Autodesk Inventor part; units mm, degrees
note: some values were not read from the file. Chosen so that the rebuilt part matches the saved one: sketch regions of "Extrusion1".
(part 2 of 2)
sketch "Sketch2" plane through (0, 0, 0) normal (0, -1, 0) x (1, 0, 0)
  line L0 (-1.935, 1.0367) -> (-1.9383, 1.036) projected
  line L1 (-1.9383, 1.036) -> (-1.9449, 1.0346) projected
  line L2 (-1.9449, 1.0346) -> (-1.9582, 1.0311) projected
  line L3 (-1.9582, 1.0311) -> (-1.9714, 1.0269) projected
  line L4 (-1.9714, 1.0269) -> (-1.9846, 1.0221) projected
  line L5 (-1.9846, 1.0221) -> (-1.9978, 1.0168) projected
  line L6 (-1.9978, 1.0168) -> (-2.0109, 1.0108) projected
  line L7 (-2.0109, 1.0108) -> (-2.0098, 0.9593) projected
  line L8 (-2.0098, 0.9593) -> (-1.9964, 0.9539) projected
  line L9 (-1.9964, 0.9539) -> (-1.983, 0.9491) projected
  line L10 (-1.983, 0.9491) -> (-1.9696, 0.9449) projected
  line L11 (-1.9696, 0.9449) -> (-1.9562, 0.9412) projected
  line L12 (-1.9562, 0.9412) -> (-1.9429, 0.9383) projected
  line L13 (-1.9429, 0.9383) -> (-1.9362, 0.9371) projected
  line L14 (-1.9362, 0.9371) -> (-1.9329, 0.9366) projected
  line L15 (-1.9329, 0.9366) -> (-1.9296, 0.9361) projected
  line L16 (-1.9296, 0.9361) -> (-1.9237, 0.8803) projected
  line L17 (-1.9237, 0.8803) -> (-1.9268, 0.8792) projected
  line L18 (-1.9268, 0.8792) -> (-1.93, 0.878) projected
  line L19 (-1.93, 0.878) -> (-1.9363, 0.8754) projected
  line L20 (-1.9363, 0.8754) -> (-1.9487, 0.8698) projected
  line L21 (-1.9487, 0.8698) -> (-1.961, 0.8634) projected
  line L22 (-1.961, 0.8634) -> (-1.9732, 0.8565) projected
  line L23 (-1.9732, 0.8565) -> (-1.9853, 0.849) projected
  line L24 (-1.9853, 0.849) -> (-1.9973, 0.8409) projected
  line L25 (-1.9973, 0.8409) -> (-1.9876, 0.7902) projected
  line L26 (-1.9876, 0.7902) -> (-1.9735, 0.7872) projected
  line L27 (-1.9735, 0.7872) -> (-1.9595, 0.7847) projected
  line L28 (-1.9595, 0.7847) -> (-1.9455, 0.7828) projected
  line L29 (-1.9455, 0.7828) -> (-1.9317, 0.7815) projected
  line L30 (-1.9317, 0.7815) -> (-1.9181, 0.7808) projected
  line L31 (-1.9181, 0.7808) -> (-1.9113, 0.7808) projected
  line L32 (-1.9113, 0.7808) -> (-1.9079, 0.7808) projected
  line L33 (-1.9079, 0.7808) -> (-1.9046, 0.7809) projected
  line L34 (-1.9046, 0.7809) -> (-1.8893, 0.727) projected
  line L35 (-1.8893, 0.727) -> (-1.8923, 0.7253) projected
  line L36 (-1.8923, 0.7253) -> (-1.8952, 0.7236) projected
  line L37 (-1.8952, 0.7236) -> (-1.9009, 0.72) projected
  line L38 (-1.9009, 0.72) -> (-1.9122, 0.7123) projected
  line L39 (-1.9122, 0.7123) -> (-1.9233, 0.704) projected
  line L40 (-1.9233, 0.704) -> (-1.9342, 0.6951) projected
  line L41 (-1.9342, 0.6951) -> (-1.9448, 0.6856) projected
  line L42 (-1.9448, 0.6856) -> (-1.9553, 0.6757) projected
  line L43 (-1.9553, 0.6757) -> (-1.9371, 0.6273) projected
  line L44 (-1.9371, 0.6273) -> (-1.9226, 0.6267) projected
  line L45 (-1.9226, 0.6267) -> (-1.9084, 0.6267) projected
  line L46 (-1.9084, 0.6267) -> (-1.8944, 0.6271) projected
  line L47 (-1.8944, 0.6271) -> (-1.8805, 0.6282) projected
  line L48 (-1.8805, 0.6282) -> (-1.8669, 0.6298) projected
  line L49 (-1.8669, 0.6298) -> (-1.8603, 0.6309) projected
  line L50 (-1.8603, 0.6309) -> (-1.857, 0.6316) projected
  line L51 (-1.857, 0.6316) -> (-1.8537, 0.6322) projected
  line L52 (-1.8537, 0.6322) -> (-1.8295, 0.5816) projected
  line L53 (-1.8295, 0.5816) -> (-1.8321, 0.5795) projected
  line L54 (-1.8321, 0.5795) -> (-1.8347, 0.5773) projected
  line L55 (-1.8347, 0.5773) -> (-1.8397, 0.5728) projected
  line L56 (-1.8397, 0.5728) -> (-1.8496, 0.5633) projected
  line L57 (-1.8496, 0.5633) -> (-1.8591, 0.5532) projected
  line L58 (-1.8591, 0.5532) -> (-1.8683, 0.5426) projected
  line L59 (-1.8683, 0.5426) -> (-1.8772, 0.5315) projected
  line L60 (-1.8772, 0.5315) -> (-1.8858, 0.5199) projected
  line L61 (-1.8858, 0.5199) -> (-1.8597, 0.4753) projected
  line L62 (-1.8597, 0.4753) -> (-1.8454, 0.4772) projected
  line L63 (-1.8454, 0.4772) -> (-1.8314, 0.4795) projected
  line L64 (-1.8314, 0.4795) -> (-1.8176, 0.4823) projected
  line L65 (-1.8176, 0.4823) -> (-1.8042, 0.4857) projected
  line L66 (-1.8042, 0.4857) -> (-1.7911, 0.4896) projected
  line L67 (-1.7911, 0.4896) -> (-1.7847, 0.4919) projected
  line L68 (-1.7847, 0.4919) -> (-1.7815, 0.493) projected
  line L69 (-1.7815, 0.493) -> (-1.7784, 0.4942) projected
  line L70 (-1.7784, 0.4942) -> (-1.746, 0.4484) projected
  line L71 (-1.746, 0.4484) -> (-1.7482, 0.4459) projected
  line L72 (-1.7482, 0.4459) -> (-1.7504, 0.4433) projected
  line L73 (-1.7504, 0.4433) -> (-1.7546, 0.438) projected
  line L74 (-1.7546, 0.438) -> (-1.7627, 0.427) projected
  line L75 (-1.7627, 0.427) -> (-1.7704, 0.4154) projected
  line L76 (-1.7704, 0.4154) -> (-1.7776, 0.4034) projected
  line L77 (-1.7776, 0.4034) -> (-1.7845, 0.391) projected
  line L78 (-1.7845, 0.391) -> (-1.7911, 0.3781) projected
  line L79 (-1.7911, 0.3781) -> (-1.7578, 0.3386) projected
  line L80 (-1.7578, 0.3386) -> (-1.744, 0.3428) projected
  line L81 (-1.744, 0.3428) -> (-1.7306, 0.3475) projected
  line L82 (-1.7306, 0.3475) -> (-1.7175, 0.3526) projected
  line L83 (-1.7175, 0.3526) -> (-1.7048, 0.3582) projected
  line L84 (-1.7048, 0.3582) -> (-1.6926, 0.3643) projected
  line L85 (-1.6926, 0.3643) -> (-1.6866, 0.3676) projected
  line L86 (-1.6866, 0.3676) -> (-1.6837, 0.3692) projected
  line L87 (-1.6837, 0.3692) -> (-1.6808, 0.371) projected
  line L88 (-1.6808, 0.371) -> (-1.6412, 0.3313) projected
  line L89 (-1.6412, 0.3313) -> (-1.6429, 0.3284) projected
  line L90 (-1.6429, 0.3284) -> (-1.6446, 0.3255) projected
  line L91 (-1.6446, 0.3255) -> (-1.6479, 0.3196) projected
  line L92 (-1.6479, 0.3196) -> (-1.654, 0.3073) projected
  line L93 (-1.654, 0.3073) -> (-1.6596, 0.2947) projected
  line L94 (-1.6596, 0.2947) -> (-1.6648, 0.2816) projected
  line L95 (-1.6648, 0.2816) -> (-1.6695, 0.2681) projected
  line L96 (-1.6695, 0.2681) -> (-1.6737, 0.2543) projected
  line L97 (-1.6737, 0.2543) -> (-1.6343, 0.221) projected
  line L98 (-1.6343, 0.221) -> (-1.6214, 0.2275) projected
  line L99 (-1.6214, 0.2275) -> (-1.6089, 0.2344) projected
  line L100 (-1.6089, 0.2344) -> (-1.5969, 0.2417) projected
  line L101 (-1.5969, 0.2417) -> (-1.5853, 0.2493) projected
  line L102 (-1.5853, 0.2493) -> (-1.5743, 0.2574) projected
  line L103 (-1.5743, 0.2574) -> (-1.569, 0.2616) projected
  line L104 (-1.569, 0.2616) -> (-1.5664, 0.2638) projected
  line L105 (-1.5664, 0.2638) -> (-1.5639, 0.266) projected
  line L106 (-1.5639, 0.266) -> (-1.5181, 0.2335) projected
  line L107 (-1.5181, 0.2335) -> (-1.5193, 0.2304) projected
  line L108 (-1.5193, 0.2304) -> (-1.5205, 0.2273) projected
  line L109 (-1.5205, 0.2273) -> (-1.5227, 0.2209) projected
  line L110 (-1.5227, 0.2209) -> (-1.5267, 0.2078) projected
  line L111 (-1.5267, 0.2078) -> (-1.5301, 0.1943) projected
  line L112 (-1.5301, 0.1943) -> (-1.5329, 0.1806) projected
  line L113 (-1.5329, 0.1806) -> (-1.5353, 0.1665) projected
  line L114 (-1.5353, 0.1665) -> (-1.5372, 0.1522) projected
  line L115 (-1.5372, 0.1522) -> (-1.4927, 0.126) projected
  line L116 (-1.4927, 0.126) -> (-1.4811, 0.1346) projected
  line L117 (-1.4811, 0.1346) -> (-1.4699, 0.1435) projected
  line L118 (-1.4699, 0.1435) -> (-1.4593, 0.1527) projected
  line L119 (-1.4593, 0.1527) -> (-1.4492, 0.1622) projected
  line L120 (-1.4492, 0.1622) -> (-1.4397, 0.172) projected
  line L121 (-1.4397, 0.172) -> (-1.4352, 0.1771) projected
  line L122 (-1.4352, 0.1771) -> (-1.433, 0.1796) projected
  line L123 (-1.433, 0.1796) -> (-1.4309, 0.1822) projected
  line L124 (-1.4309, 0.1822) -> (-1.3803, 0.158) projected
  line L125 (-1.3803, 0.158) -> (-1.3809, 0.1547) projected
  line L126 (-1.3809, 0.1547) -> (-1.3816, 0.1514) projected
  line L127 (-1.3816, 0.1514) -> (-1.3827, 0.1447) projected
  line L128 (-1.3827, 0.1447) -> (-1.3844, 0.1312) projected
  line L129 (-1.3844, 0.1312) -> (-1.3854, 0.1173) projected
  line L130 (-1.3854, 0.1173) -> (-1.3859, 0.1033) projected
  line L131 (-1.3859, 0.1033) -> (-1.3859, 0.089) projected
  line L132 (-1.3859, 0.089) -> (-1.3853, 0.0746) projected
  line L133 (-1.3853, 0.0746) -> (-1.337, 0.0563) projected
  line L134 (-1.337, 0.0563) -> (-1.327, 0.0668) projected
  line L135 (-1.327, 0.0668) -> (-1.3176, 0.0774) projected
  line L136 (-1.3176, 0.0774) -> (-1.3086, 0.0883) projected
  line L137 (-1.3086, 0.0883) -> (-1.3003, 0.0993) projected
  line L138 (-1.3003, 0.0993) -> (-1.2926, 0.1106) projected
  line L139 (-1.2926, 0.1106) -> (-1.289, 0.1164) projected
  line L140 (-1.289, 0.1164) -> (-1.2873, 0.1193) projected
  line L141 (-1.2873, 0.1193) -> (-1.2856, 0.1222) projected
  line L142 (-1.2856, 0.1222) -> (-1.2316, 0.1068) projected
  line L143 (-1.2316, 0.1068) -> (-1.2318, 0.1035) projected
  line L144 (-1.2318, 0.1035) -> (-1.2318, 0.1001) projected
  line L145 (-1.2318, 0.1001) -> (-1.2318, 0.0934) projected
  line L146 (-1.2318, 0.0934) -> (-1.2312, 0.0797) projected
  line L147 (-1.2312, 0.0797) -> (-1.2299, 0.0659) projected
  line L148 (-1.2299, 0.0659) -> (-1.228, 0.052) projected
  line L149 (-1.228, 0.052) -> (-1.2255, 0.0379) projected
  line L150 (-1.2255, 0.0379) -> (-1.2225, 0.0238) projected
  line L151 (-1.2225, 0.0238) -> (-1.1718, 0.014) projected
  line L152 (-1.1718, 0.014) -> (-1.1638, 0.0259) projected
  line L153 (-1.1638, 0.0259) -> (-1.1562, 0.038) projected
  line L154 (-1.1562, 0.038) -> (-1.1492, 0.0502) projected
  line L155 (-1.1492, 0.0502) -> (-1.1429, 0.0625) projected
  line L156 (-1.1429, 0.0625) -> (-1.1372, 0.075) projected
  line L157 (-1.1372, 0.075) -> (-1.1346, 0.0812) projected
  line L158 (-1.1346, 0.0812) -> (-1.1334, 0.0844) projected
  line L159 (-1.1334, 0.0844) -> (-1.1323, 0.0875) projected
  line L160 (-1.1323, 0.0875) -> (-1.0765, 0.0815) projected
  line L161 (-1.0765, 0.0815) -> (-1.076, 0.0782) projected
  line L162 (-1.076, 0.0782) -> (-1.0755, 0.0749) projected
  line L163 (-1.0755, 0.0749) -> (-1.0744, 0.0682) projected
  line L164 (-1.0744, 0.0682) -> (-1.0714, 0.0548) projected
  line L165 (-1.0714, 0.0548) -> (-1.0678, 0.0415) projected
  line L166 (-1.0678, 0.0415) -> (-1.0636, 0.028) projected
  line L167 (-1.0636, 0.028) -> (-1.0588, 0.0146) projected
  line L168 (-1.0588, 0.0146) -> (-1.0535, 0.0012) projected
  line L169 (-1.0535, 0.0012) -> (-1.0019, 0.0001) projected
  line L170 (-1.0019, 0.0001) -> (-0.9959, 0.0132) projected
  line L171 (-0.9959, 0.0132) -> (-0.9905, 0.0264) projected
  line L172 (-0.9905, 0.0264) -> (-0.9857, 0.0396) projected
  line L173 (-0.9857, 0.0396) -> (-0.9815, 0.0528) projected
  line L174 (-0.9815, 0.0528) -> (-0.978, 0.0661) projected
  line L175 (-0.978, 0.0661) -> (-0.9765, 0.0727) projected
  line L176 (-0.9765, 0.0727) -> (-0.9759, 0.076) projected
  line L177 (-0.9759, 0.076) -> (-0.9753, 0.0793) projected
  line L178 (-0.9753, 0.0793) -> (-0.9193, 0.0828) projected
  line L179 (-0.9193, 0.0828) -> (-0.9183, 0.0796) projected
  line L180 (-0.9183, 0.0796) -> (-0.9172, 0.0764) projected
  line L181 (-0.9172, 0.0764) -> (-0.9149, 0.07) projected
  line L182 (-0.9149, 0.07) -> (-0.9098, 0.0573) projected
  line L183 (-0.9098, 0.0573) -> (-0.904, 0.0448) projected
  line L184 (-0.904, 0.0448) -> (-0.8976, 0.0323) projected
  line L185 (-0.8976, 0.0323) -> (-0.8906, 0.0198) projected
  line L186 (-0.8906, 0.0198) -> (-0.883, 0.0075) projected
  line L187 (-0.883, 0.0075) -> (-0.832, 0.0151) projected
  line L188 (-0.832, 0.0151) -> (-0.8284, 0.0291) projected
  line L189 (-0.8284, 0.0291) -> (-0.8253, 0.043) projected
  line L190 (-0.8253, 0.043) -> (-0.8228, 0.0568) projected
  line L191 (-0.8228, 0.0568) -> (-0.8209, 0.0706) projected
  line L192 (-0.8209, 0.0706) -> (-0.8197, 0.0842) projected
  line L193 (-0.8197, 0.0842) -> (-0.8193, 0.0909) projected
  line L194 (-0.8193, 0.0909) -> (-0.8192, 0.0943) projected
  line L195 (-0.8192, 0.0943) -> (-0.8192, 0.0977) projected
  line L196 (-0.8192, 0.0977) -> (-0.7646, 0.1106) projected
  line L197 (-0.7646, 0.1106) -> (-0.7631, 0.1076) projected
  line L198 (-0.7631, 0.1076) -> (-0.7615, 0.1046) projected
  line L199 (-0.7615, 0.1046) -> (-0.7581, 0.0987) projected
  line L200 (-0.7581, 0.0987) -> (-0.751, 0.0871) projected
  line L201 (-0.751, 0.0871) -> (-0.7431, 0.0757) projected
  line L202 (-0.7431, 0.0757) -> (-0.7347, 0.0645) projected
  line L203 (-0.7347, 0.0645) -> (-0.7257, 0.0534) projected
  line L204 (-0.7257, 0.0534) -> (-0.7161, 0.0426) projected
  line L205 (-0.7161, 0.0426) -> (-0.6671, 0.0587) projected
  line L206 (-0.6671, 0.0587) -> (-0.6659, 0.0731) projected
  line L207 (-0.6659, 0.0731) -> (-0.6652, 0.0873) projected
  line L208 (-0.6652, 0.0873) -> (-0.6651, 0.1013) projected
  line L209 (-0.6651, 0.1013) -> (-0.6655, 0.1152) projected
  line L210 (-0.6655, 0.1152) -> (-0.6666, 0.1288) projected
  line L211 (-0.6666, 0.1288) -> (-0.6674, 0.1355) projected
  line L212 (-0.6674, 0.1355) -> (-0.6679, 0.1389) projected
  line L213 (-0.6679, 0.1389) -> (-0.6684, 0.1422) projected
  line L214 (-0.6684, 0.1422) -> (-0.6168, 0.1641) projected
  line L215 (-0.6168, 0.1641) -> (-0.6148, 0.1615) projected
  line L216 (-0.6148, 0.1615) -> (-0.6127, 0.1588) projected
  line L217 (-0.6127, 0.1588) -> (-0.6085, 0.1536) projected
  line L218 (-0.6085, 0.1536) -> (-0.5994, 0.1433) projected
  line L219 (-0.5994, 0.1433) -> (-0.5897, 0.1334) projected
  line L220 (-0.5897, 0.1334) -> (-0.5795, 0.1238) projected
  line L221 (-0.5795, 0.1238) -> (-0.5688, 0.1144) projected
  line L222 (-0.5688, 0.1144) -> (-0.5576, 0.1053) projected
  line L223 (-0.5576, 0.1053) -> (-0.512, 0.1294) projected
  line L224 (-0.512, 0.1294) -> (-0.5132, 0.1438) projected
  line L225 (-0.5132, 0.1438) -> (-0.5149, 0.158) projected
  line L226 (-0.5149, 0.158) -> (-0.5172, 0.1718) projected
  line L227 (-0.5172, 0.1718) -> (-0.5199, 0.1854) projected
  line L228 (-0.5199, 0.1854) -> (-0.5233, 0.1987) projected
  line L229 (-0.5233, 0.1987) -> (-0.5253, 0.2052) projected
  line L230 (-0.5253, 0.2052) -> (-0.5263, 0.2084) projected
  line L231 (-0.5263, 0.2084) -> (-0.5274, 0.2115) projected
  line L232 (-0.5274, 0.2115) -> (-0.4802, 0.2419) projected
  line L233 (-0.4802, 0.2419) -> (-0.4778, 0.2396) projected
  line L234 (-0.4778, 0.2396) -> (-0.4753, 0.2373) projected
  line L235 (-0.4753, 0.2373) -> (-0.4702, 0.2329) projected
  line L236 (-0.4702, 0.2329) -> (-0.4595, 0.2243) projected
  line L237 (-0.4595, 0.2243) -> (-0.4483, 0.2162) projected
  line L238 (-0.4483, 0.2162) -> (-0.4366, 0.2084) projected
  line L239 (-0.4366, 0.2084) -> (-0.4244, 0.201) projected
  line L240 (-0.4244, 0.201) -> (-0.4119, 0.1939) projected
  line L241 (-0.4119, 0.1939) -> (-0.371, 0.2254) projected
  line L242 (-0.371, 0.2254) -> (-0.3746, 0.2394) projected
  line L243 (-0.3746, 0.2394) -> (-0.3787, 0.2531) projected
  line L244 (-0.3787, 0.2531) -> (-0.3833, 0.2664) projected
  line L245 (-0.3833, 0.2664) -> (-0.3883, 0.2793) projected
  line L246 (-0.3883, 0.2793) -> (-0.3939, 0.2918) projected
  line L247 (-0.3939, 0.2918) -> (-0.3969, 0.2978) projected
  line L248 (-0.3969, 0.2978) -> (-0.3985, 0.3008) projected
  line L249 (-0.3985, 0.3008) -> (-0.4001, 0.3037) projected
  line L250 (-0.4001, 0.3037) -> (-0.3587, 0.3417) projected
  line L251 (-0.3587, 0.3417) -> (-0.3559, 0.3398) projected
  line L252 (-0.3559, 0.3398) -> (-0.3531, 0.338) projected
  line L253 (-0.3531, 0.338) -> (-0.3473, 0.3345) projected
  line L254 (-0.3473, 0.3345) -> (-0.3354, 0.3278) projected
  line L255 (-0.3354, 0.3278) -> (-0.3229, 0.3217) projected
  line L256 (-0.3229, 0.3217) -> (-0.3101, 0.316) projected
  line L257 (-0.3101, 0.316) -> (-0.2969, 0.3108) projected
  line L258 (-0.2969, 0.3108) -> (-0.2832, 0.3059) projected
  line L259 (-0.2832, 0.3059) -> (-0.2483, 0.3439) projected
  line L260 (-0.2483, 0.3439) -> (-0.2543, 0.357) projected
  line L261 (-0.2543, 0.357) -> (-0.2606, 0.3698) projected
  line L262 (-0.2606, 0.3698) -> (-0.2673, 0.3821) projected
  line L263 (-0.2673, 0.3821) -> (-0.2745, 0.394) projected
  line L264 (-0.2745, 0.394) -> (-0.2821, 0.4054) projected
  line L265 (-0.2821, 0.4054) -> (-0.2861, 0.4108) projected
  line L266 (-0.2861, 0.4108) -> (-0.2881, 0.4135) projected
  line L267 (-0.2881, 0.4135) -> (-0.2902, 0.4161) projected
  line L268 (-0.2902, 0.4161) -> (-0.2559, 0.4605) projected
  line L269 (-0.2559, 0.4605) -> (-0.2528, 0.4592) projected
  line L270 (-0.2528, 0.4592) -> (-0.2497, 0.4578) projected
  line L271 (-0.2497, 0.4578) -> (-0.2434, 0.4553) projected
  line L272 (-0.2434, 0.4553) -> (-0.2305, 0.4508) projected
  line L273 (-0.2305, 0.4508) -> (-0.2172, 0.4469) projected
  line L274 (-0.2172, 0.4469) -> (-0.2036, 0.4434) projected
  line L275 (-0.2036, 0.4434) -> (-0.1896, 0.4405) projected
  line L276 (-0.1896, 0.4405) -> (-0.1754, 0.438) projected
  line L277 (-0.1754, 0.438) -> (-0.1474, 0.4814) projected
  line L278 (-0.1474, 0.4814) -> (-0.1555, 0.4933) projected
  line L279 (-0.1555, 0.4933) -> (-0.1639, 0.5048) projected
  line L280 (-0.1639, 0.5048) -> (-0.1726, 0.5158) projected
  line L281 (-0.1726, 0.5158) -> (-0.1817, 0.5263) projected
  line L282 (-0.1817, 0.5263) -> (-0.1911, 0.5363) projected
  line L283 (-0.1911, 0.5363) -> (-0.1959, 0.541) projected
  line L284 (-0.1959, 0.541) -> (-0.1984, 0.5433) projected
  line L285 (-0.1984, 0.5433) -> (-0.2009, 0.5455) projected
  line L286 (-0.2009, 0.5455) -> (-0.1745, 0.595) projected
  line L287 (-0.1745, 0.595) -> (-0.1713, 0.5942) projected
  line L288 (-0.1713, 0.5942) -> (-0.168, 0.5934) projected
  line L289 (-0.168, 0.5934) -> (-0.1614, 0.592) projected
  line L290 (-0.1614, 0.592) -> (-0.1479, 0.5898) projected
  line L291 (-0.1479, 0.5898) -> (-0.1341, 0.5881) projected
  line L292 (-0.1341, 0.5881) -> (-0.1201, 0.587) projected
  line L293 (-0.1201, 0.587) -> (-0.1059, 0.5865) projected
  line L294 (-0.1059, 0.5865) -> (-0.0915, 0.5865) projected
  line L295 (-0.0915, 0.5865) -> (-0.0712, 0.6339) projected
  line L296 (-0.0712, 0.6339) -> (-0.0812, 0.6443) projected
  line L297 (-0.0812, 0.6443) -> (-0.0914, 0.6543) projected
  line L298 (-0.0914, 0.6543) -> (-0.1018, 0.6636) projected
  line L299 (-0.1018, 0.6636) -> (-0.1125, 0.6725) projected
  line L300 (-0.1125, 0.6725) -> (-0.1235, 0.6806) projected
  line L301 (-0.1235, 0.6806) -> (-0.1291, 0.6845) projected
  line L302 (-0.1291, 0.6845) -> (-0.1319, 0.6863) projected
  line L303 (-0.1319, 0.6863) -> (-0.1347, 0.6881) projected
  line L304 (-0.1347, 0.6881) -> (-0.1171, 0.7414) projected
  line L305 (-0.1171, 0.7414) -> (-0.1138, 0.7411) projected
  line L306 (-0.1138, 0.7411) -> (-0.1104, 0.7409) projected
  line L307 (-0.1104, 0.7409) -> (-0.1037, 0.7406) projected
  line L308 (-0.1037, 0.7406) -> (-0.09, 0.7407) projected
  line L309 (-0.09, 0.7407) -> (-0.0761, 0.7414) projected
  line L310 (-0.0761, 0.7414) -> (-0.0621, 0.7427) projected
  line L311 (-0.0621, 0.7427) -> (-0.048, 0.7446) projected
  line L312 (-0.048, 0.7446) -> (-0.0338, 0.747) projected
  line L313 (-0.0338, 0.747) -> (-0.0218, 0.7972) projected
  line L314 (-0.0218, 0.7972) -> (-0.0334, 0.8057) projected
  line L315 (-0.0334, 0.8057) -> (-0.0452, 0.8138) projected
  line L316 (-0.0452, 0.8138) -> (-0.0571, 0.8213) projected
  line L317 (-0.0571, 0.8213) -> (-0.0691, 0.8282) projected
  line L318 (-0.0691, 0.8282) -> (-0.0813, 0.8344) projected
  line L319 (-0.0813, 0.8344) -> (-0.0874, 0.8372) projected
  line L320 (-0.0874, 0.8372) -> (-0.0905, 0.8385) projected
  line L321 (-0.0905, 0.8385) -> (-0.0936, 0.8398) projected
  line L322 (-0.0936, 0.8398) -> (-0.0853, 0.8953) projected
  line L323 (-0.0853, 0.8953) -> (-0.0819, 0.8956) projected
  line L324 (-0.0819, 0.8956) -> (-0.0786, 0.896) projected
  line L325 (-0.0786, 0.896) -> (-0.0719, 0.8969) projected
  line L326 (-0.0719, 0.8969) -> (-0.0584, 0.8992) projected
  line L327 (-0.0584, 0.8992) -> (-0.0449, 0.9022) projected
  line L328 (-0.0449, 0.9022) -> (-0.0313, 0.9059) projected
  line L329 (-0.0313, 0.9059) -> (-0.0177, 0.9101) projected
  line L330 (-0.0177, 0.9101) -> (-0.0041, 0.9149) projected
  line L331 (-0.0041, 0.9149) -> (-0.0008, 0.9664) projected
  line L332 (-0.0008, 0.9664) -> (-0.0137, 0.9729) projected
  line L333 (-0.0137, 0.9729) -> (-0.0266, 0.9788) projected
  line L334 (-0.0266, 0.9788) -> (-0.0396, 0.9842) projected
  line L335 (-0.0396, 0.9842) -> (-0.0526, 0.9889) projected
  line L336 (-0.0526, 0.9889) -> (-0.0657, 0.993) projected
  line L337 (-0.0657, 0.993) -> (-0.0722, 0.9948) projected
  line L338 (-0.0722, 0.9948) -> (-0.0755, 0.9955) projected
  line L339 (-0.0755, 0.9955) -> (-0.0788, 0.9963) projected
  line L340 (-0.0788, 0.9963) -> (-0.0799, 1.0524) projected
  line L341 (-0.0799, 1.0524) -> (-0.0767, 1.0533) projected
  line L342 (-0.0767, 1.0533) -> (-0.0734, 1.0542) projected
  line L343 (-0.0734, 1.0542) -> (-0.067, 1.0562) projected
  line L344 (-0.067, 1.0562) -> (-0.0541, 1.0608) projected
  line L345 (-0.0541, 1.0608) -> (-0.0413, 1.0661) projected
  line L346 (-0.0413, 1.0661) -> (-0.0285, 1.072) projected
  line L347 (-0.0285, 1.072) -> (-0.0158, 1.0784) projected
  line L348 (-0.0158, 1.0784) -> (-0.0032, 1.0854) projected
  line L349 (-0.0032, 1.0854) -> (-0.0086, 1.1368) projected
  line L350 (-0.0086, 1.1368) -> (-0.0224, 1.141) projected
  line L351 (-0.0224, 1.141) -> (-0.0362, 1.1446) projected
  line L352 (-0.0362, 1.1446) -> (-0.0499, 1.1477) projected
  line L353 (-0.0499, 1.1477) -> (-0.0635, 1.1502) projected
  line L354 (-0.0635, 1.1502) -> (-0.0771, 1.152) projected
  line L355 (-0.0771, 1.152) -> (-0.0838, 1.1526) projected
  line L356 (-0.0838, 1.1526) -> (-0.0872, 1.1529) projected
  line L357 (-0.0872, 1.1529) -> (-0.0905, 1.153) projected
  line L358 (-0.0905, 1.153) -> (-0.1011, 1.2081) projected
  line L359 (-0.1011, 1.2081) -> (-0.0981, 1.2095) projected
  line L360 (-0.0981, 1.2095) -> (-0.0951, 1.211) projected
  line L361 (-0.0951, 1.211) -> (-0.089, 1.2141) projected
  line L362 (-0.089, 1.2141) -> (-0.0771, 1.2208) projected
  line L363 (-0.0771, 1.2208) -> (-0.0654, 1.2281) projected
  line L364 (-0.0654, 1.2281) -> (-0.0538, 1.2361) projected
  line L365 (-0.0538, 1.2361) -> (-0.0424, 1.2446) projected
  line L366 (-0.0424, 1.2446) -> (-0.0311, 1.2537) projected
  line L367 (-0.0311, 1.2537) -> (-0.0451, 1.3033) projected
  line L368 (-0.0451, 1.3033) -> (-0.0595, 1.3052) projected
  line L369 (-0.0595, 1.3052) -> (-0.0736, 1.3065) projected
  line L370 (-0.0736, 1.3065) -> (-0.0877, 1.3072) projected
  line L371 (-0.0877, 1.3072) -> (-0.1015, 1.3073) projected
  line L372 (-0.1015, 1.3073) -> (-0.1152, 1.3068) projected
  line L373 (-0.1152, 1.3068) -> (-0.122, 1.3063) projected
  line L374 (-0.122, 1.3063) -> (-0.1253, 1.3059) projected
  line L375 (-0.1253, 1.3059) -> (-0.1286, 1.3055) projected
  line L376 (-0.1286, 1.3055) -> (-0.1484, 1.358) projected
  line L377 (-0.1484, 1.358) -> (-0.1456, 1.3599) projected
  line L378 (-0.1456, 1.3599) -> (-0.1429, 1.3619) projected
  line L379 (-0.1429, 1.3619) -> (-0.1375, 1.3659) projected
  line L380 (-0.1375, 1.3659) -> (-0.1269, 1.3746) projected
  line L381 (-0.1269, 1.3746) -> (-0.1165, 1.3838) projected
  line L382 (-0.1165, 1.3838) -> (-0.1065, 1.3936) projected
  line L383 (-0.1065, 1.3936) -> (-0.0966, 1.4039) projected
  line L384 (-0.0966, 1.4039) -> (-0.0871, 1.4148) projected
  line L385 (-0.0871, 1.4148) -> (-0.1093, 1.4613) projected
  line L386 (-0.1093, 1.4613) -> (-0.1237, 1.4607) projected
  line L387 (-0.1237, 1.4607) -> (-0.1379, 1.4596) projected
  line L388 (-0.1379, 1.4596) -> (-0.1519, 1.458) projected
  line L389 (-0.1519, 1.458) -> (-0.1656, 1.4557) projected
  line L390 (-0.1656, 1.4557) -> (-0.1789, 1.4529) projected
  line L391 (-0.1789, 1.4529) -> (-0.1855, 1.4513) projected
  line L392 (-0.1855, 1.4513) -> (-0.1887, 1.4504) projected
  line L393 (-0.1887, 1.4504) -> (-0.192, 1.4494) projected
  line L394 (-0.192, 1.4494) -> (-0.2203, 1.4978) projected
  line L395 (-0.2203, 1.4978) -> (-0.2179, 1.5002) projected
  line L396 (-0.2179, 1.5002) -> (-0.2155, 1.5025) projected
  line L397 (-0.2155, 1.5025) -> (-0.2109, 1.5075) projected
  line L398 (-0.2109, 1.5075) -> (-0.2019, 1.5177) projected
  line L399 (-0.2019, 1.5177) -> (-0.1933, 1.5286) projected
  line L400 (-0.1933, 1.5286) -> (-0.185, 1.54) projected
  line L401 (-0.185, 1.54) -> (-0.1771, 1.5518) projected
  line L402 (-0.1771, 1.5518) -> (-0.1695, 1.5641) projected
  line L403 (-0.1695, 1.5641) -> (-0.1992, 1.6062) projected
  line L404 (-0.1992, 1.6062) -> (-0.2133, 1.6032) projected
  line L405 (-0.2133, 1.6032) -> (-0.2271, 1.5997) projected
  line L406 (-0.2271, 1.5997) -> (-0.2406, 1.5957) projected
  line L407 (-0.2406, 1.5957) -> (-0.2537, 1.5912) projected
  line L408 (-0.2537, 1.5912) -> (-0.2665, 1.5862) projected
  line L409 (-0.2665, 1.5862) -> (-0.2726, 1.5834) projected
  line L410 (-0.2726, 1.5834) -> (-0.2757, 1.582) projected
  line L411 (-0.2757, 1.582) -> (-0.2787, 1.5805) projected
  line L412 (-0.2787, 1.5805) -> (-0.3148, 1.6234) projected
  line L413 (-0.3148, 1.6234) -> (-0.3128, 1.6261) projected
  line L414 (-0.3128, 1.6261) -> (-0.3109, 1.6289) projected
  line L415 (-0.3109, 1.6289) -> (-0.3071, 1.6345) projected
  line L416 (-0.3071, 1.6345) -> (-0.3, 1.6462) projected
  line L417 (-0.3, 1.6462) -> (-0.2933, 1.6583) projected
  line L418 (-0.2933, 1.6583) -> (-0.2871, 1.6709) projected
  line L419 (-0.2871, 1.6709) -> (-0.2813, 1.6839) projected
  line L420 (-0.2813, 1.6839) -> (-0.2759, 1.6973) projected
  line L421 (-0.2759, 1.6973) -> (-0.3123, 1.7339) projected
  line L422 (-0.3123, 1.7339) -> (-0.3257, 1.7285) projected
  line L423 (-0.3257, 1.7285) -> (-0.3388, 1.7227) projected
  line L424 (-0.3388, 1.7227) -> (-0.3514, 1.7165) projected
  line L425 (-0.3514, 1.7165) -> (-0.3635, 1.7098) projected
  line L426 (-0.3635, 1.7098) -> (-0.3752, 1.7027) projected
  line L427 (-0.3752, 1.7027) -> (-0.3809, 1.699) projected
  line L428 (-0.3809, 1.699) -> (-0.3836, 1.697) projected
  line L429 (-0.3836, 1.697) -> (-0.3863, 1.6951) projected
  line L430 (-0.3863, 1.6951) -> (-0.4292, 1.7313) projected
  line L431 (-0.4292, 1.7313) -> (-0.4277, 1.7343) projected
  line L432 (-0.4277, 1.7343) -> (-0.4263, 1.7373) projected
  line L433 (-0.4263, 1.7373) -> (-0.4235, 1.7435) projected
  line L434 (-0.4235, 1.7435) -> (-0.4184, 1.7562) projected
  line L435 (-0.4184, 1.7562) -> (-0.4139, 1.7693) projected
  line L436 (-0.4139, 1.7693) -> (-0.4099, 1.7828) projected
  line L437 (-0.4099, 1.7828) -> (-0.4064, 1.7966) projected
  line L438 (-0.4064, 1.7966) -> (-0.4033, 1.8107) projected
  line L439 (-0.4033, 1.8107) -> (-0.4454, 1.8405) projected
  line L440 (-0.4454, 1.8405) -> (-0.4577, 1.8329) projected
  line L441 (-0.4577, 1.8329) -> (-0.4696, 1.825) projected
  line L442 (-0.4696, 1.825) -> (-0.4809, 1.8168) projected
  line L443 (-0.4809, 1.8168) -> (-0.4918, 1.8082) projected
  line L444 (-0.4918, 1.8082) -> (-0.5021, 1.7992) projected
  line L445 (-0.5021, 1.7992) -> (-0.507, 1.7945) projected
  line L446 (-0.507, 1.7945) -> (-0.5094, 1.7922) projected
  line L447 (-0.5094, 1.7922) -> (-0.5118, 1.7898) projected
  line L448 (-0.5118, 1.7898) -> (-0.5601, 1.8182) projected
  line L449 (-0.5601, 1.8182) -> (-0.5592, 1.8214) projected
  line L450 (-0.5592, 1.8214) -> (-0.5583, 1.8247) projected
  line L451 (-0.5583, 1.8247) -> (-0.5566, 1.8312) projected
  line L452 (-0.5566, 1.8312) -> (-0.5537, 1.8446) projected
  line L453 (-0.5537, 1.8446) -> (-0.5515, 1.8583) projected
  line L454 (-0.5515, 1.8583) -> (-0.5498, 1.8722) projected
  line L455 (-0.5498, 1.8722) -> (-0.5487, 1.8864) projected
  line L456 (-0.5487, 1.8864) -> (-0.548, 1.9009) projected
  line L457 (-0.548, 1.9009) -> (-0.5946, 1.9232) projected
  line L458 (-0.5946, 1.9232) -> (-0.6054, 1.9136) projected
  line L459 (-0.6054, 1.9136) -> (-0.6158, 1.9038) projected
  line L460 (-0.6158, 1.9038) -> (-0.6256, 1.8938) projected
  line L461 (-0.6256, 1.8938) -> (-0.6349, 1.8834) projected
  line L462 (-0.6349, 1.8834) -> (-0.6435, 1.8728) projected
  line L463 (-0.6435, 1.8728) -> (-0.6476, 1.8674) projected
  line L464 (-0.6476, 1.8674) -> (-0.6495, 1.8647) projected
  line L465 (-0.6495, 1.8647) -> (-0.6514, 1.8619) projected
  line L466 (-0.6514, 1.8619) -> (-0.7039, 1.8818) projected
  line L467 (-0.7039, 1.8818) -> (-0.7035, 1.8851) projected
  line L468 (-0.7035, 1.8851) -> (-0.7031, 1.8885) projected
  line L469 (-0.7031, 1.8885) -> (-0.7026, 1.8952) projected
  line L470 (-0.7026, 1.8952) -> (-0.7021, 1.9089) projected
  line L471 (-0.7021, 1.9089) -> (-0.7022, 1.9227) projected
  line L472 (-0.7022, 1.9227) -> (-0.7029, 1.9368) projected
  line L473 (-0.7029, 1.9368) -> (-0.7041, 1.951) projected
  line L474 (-0.7041, 1.951) -> (-0.706, 1.9653) projected
  line L475 (-0.706, 1.9653) -> (-0.7556, 1.9794) projected
  line L476 (-0.7556, 1.9794) -> (-0.7647, 1.9682) projected
  line L477 (-0.7647, 1.9682) -> (-0.7732, 1.9567) projected
  line L478 (-0.7732, 1.9567) -> (-0.7812, 1.9452) projected
  line L479 (-0.7812, 1.9452) -> (-0.7886, 1.9334) projected
  line L480 (-0.7886, 1.9334) -> (-0.7953, 1.9215) projected
  line L481 (-0.7953, 1.9215) -> (-0.7984, 1.9155) projected
  line L482 (-0.7984, 1.9155) -> (-0.7998, 1.9125) projected
  line L483 (-0.7998, 1.9125) -> (-0.8013, 1.9094) projected
  line L484 (-0.8013, 1.9094) -> (-0.8563, 1.9201) projected
  line L485 (-0.8563, 1.9201) -> (-0.8565, 1.9235) projected
  line L486 (-0.8565, 1.9235) -> (-0.8567, 1.9268) projected
  line L487 (-0.8567, 1.9268) -> (-0.8573, 1.9336) projected
  line L488 (-0.8573, 1.9336) -> (-0.8591, 1.9471) projected
  line L489 (-0.8591, 1.9471) -> (-0.8616, 1.9608) projected
  line L490 (-0.8616, 1.9608) -> (-0.8646, 1.9745) projected
  line L491 (-0.8646, 1.9745) -> (-0.8683, 1.9883) projected
  line L492 (-0.8683, 1.9883) -> (-0.8725, 2.0021) projected
  line L493 (-0.8725, 2.0021) -> (-0.9238, 2.0076) projected
  line L494 (-0.9238, 2.0076) -> (-0.9308, 1.995) projected
  line L495 (-0.9308, 1.995) -> (-0.9373, 1.9823) projected
  line L496 (-0.9373, 1.9823) -> (-0.9432, 1.9696) projected
  line L497 (-0.9432, 1.9696) -> (-0.9485, 1.9568) projected
  line L498 (-0.9485, 1.9568) -> (-0.9531, 1.9439) projected
  line L499 (-0.9531, 1.9439) -> (-0.9552, 1.9374) projected
  line L500 (-0.9552, 1.9374) -> (-0.9561, 1.9342) projected
  line L501 (-0.9561, 1.9342) -> (-0.957, 1.931) projected
  line L502 (-0.957, 1.931) -> (-1.0131, 1.9322) projected
  line L503 (-1.0131, 1.9322) -> (-1.0138, 1.9355) projected
  line L504 (-1.0138, 1.9355) -> (-1.0146, 1.9387) projected
  line L505 (-1.0146, 1.9387) -> (-1.0163, 1.9453) projected
  line L506 (-1.0163, 1.9453) -> (-1.0203, 1.9583) projected
  line L507 (-1.0203, 1.9583) -> (-1.0251, 1.9714) projected
  line L508 (-1.0251, 1.9714) -> (-1.0304, 1.9844) projected
  line L509 (-1.0304, 1.9844) -> (-1.0363, 1.9973) projected
  line L510 (-1.0363, 1.9973) -> (-1.0428, 2.0102) projected
  line L511 (-1.0428, 2.0102) -> (-1.0943, 2.007) projected
  line L512 (-1.0943, 2.007) -> (-1.0991, 1.9934) projected
  line L513 (-1.0991, 1.9934) -> (-1.1034, 1.9798) projected
  line L514 (-1.1034, 1.9798) -> (-1.107, 1.9662) projected
  line L515 (-1.107, 1.9662) -> (-1.1101, 1.9527) projected
  line L516 (-1.1101, 1.9527) -> (-1.1125, 1.9392) projected
  line L517 (-1.1125, 1.9392) -> (-1.1134, 1.9325) projected
  line L518 (-1.1134, 1.9325) -> (-1.1138, 1.9292) projected
  line L519 (-1.1138, 1.9292) -> (-1.1141, 1.9259) projected
  line L520 (-1.1141, 1.9259) -> (-1.1696, 1.9176) projected
  line L521 (-1.1696, 1.9176) -> (-1.1708, 1.9207) projected
  line L522 (-1.1708, 1.9207) -> (-1.1722, 1.9238) projected
  line L523 (-1.1722, 1.9238) -> (-1.175, 1.9299) projected
  line L524 (-1.175, 1.9299) -> (-1.1812, 1.9421) projected
  line L525 (-1.1812, 1.9421) -> (-1.188, 1.9542) projected
  line L526 (-1.188, 1.9542) -> (-1.1955, 1.9661) projected
  line L527 (-1.1955, 1.9661) -> (-1.2035, 1.9779) projected
  line L528 (-1.2035, 1.9779) -> (-1.2121, 1.9895) projected
  line L529 (-1.2121, 1.9895) -> (-1.2623, 1.9776) projected
  line L530 (-1.2623, 1.9776) -> (-1.2647, 1.9634) projected
  line L531 (-1.2647, 1.9634) -> (-1.2666, 1.9493) projected
  line L532 (-1.2666, 1.9493) -> (-1.268, 1.9353) projected
  line L533 (-1.268, 1.9353) -> (-1.2687, 1.9214) projected
  line L534 (-1.2687, 1.9214) -> (-1.2688, 1.9077) projected
  line L535 (-1.2688, 1.9077) -> (-1.2685, 1.901) projected
  line L536 (-1.2685, 1.901) -> (-1.2683, 1.8976) projected
  line L537 (-1.2683, 1.8976) -> (-1.2681, 1.8943) projected
  line L538 (-1.2681, 1.8943) -> (-1.3214, 1.8768) projected
  line L539 (-1.3214, 1.8768) -> (-1.3231, 1.8796) projected
  line L540 (-1.3231, 1.8796) -> (-1.325, 1.8824) projected
  line L541 (-1.325, 1.8824) -> (-1.3288, 1.888) projected
  line L542 (-1.3288, 1.888) -> (-1.337, 1.899) projected
  line L543 (-1.337, 1.899) -> (-1.3458, 1.9097) projected
  line L544 (-1.3458, 1.9097) -> (-1.3551, 1.9202) projected
  line L545 (-1.3551, 1.9202) -> (-1.365, 1.9304) projected
  line L546 (-1.365, 1.9304) -> (-1.3754, 1.9405) projected
  line L547 (-1.3754, 1.9405) -> (-1.4229, 1.9202) projected
  line L548 (-1.4229, 1.9202) -> (-1.4229, 1.9058) projected
  line L549 (-1.4229, 1.9058) -> (-1.4224, 1.8916) projected
  line L550 (-1.4224, 1.8916) -> (-1.4213, 1.8776) projected
  line L551 (-1.4213, 1.8776) -> (-1.4197, 1.8638) projected
  line L552 (-1.4197, 1.8638) -> (-1.4175, 1.8503) projected
  line L553 (-1.4175, 1.8503) -> (-1.4161, 1.8437) projected
  line L554 (-1.4161, 1.8437) -> (-1.4153, 1.8404) projected
  line L555 (-1.4153, 1.8404) -> (-1.4145, 1.8371) projected
  line L556 (-1.4145, 1.8371) -> (-1.4641, 1.8109) projected
  line L557 (-1.4641, 1.8109) -> (-1.4663, 1.8134) projected
  line L558 (-1.4663, 1.8134) -> (-1.4686, 1.8158) projected
  line L559 (-1.4686, 1.8158) -> (-1.4733, 1.8207) projected
  line L560 (-1.4733, 1.8207) -> (-1.4832, 1.8301) projected
  line L561 (-1.4832, 1.8301) -> (-1.4937, 1.8392) projected
  line L562 (-1.4937, 1.8392) -> (-1.5047, 1.848) projected
  line L563 (-1.5047, 1.848) -> (-1.5162, 1.8564) projected
  line L564 (-1.5162, 1.8564) -> (-1.5281, 1.8645) projected
  line L565 (-1.5281, 1.8645) -> (-1.5715, 1.8365) projected
  line L566 (-1.5715, 1.8365) -> (-1.5691, 1.8223) projected
  line L567 (-1.5691, 1.8223) -> (-1.5661, 1.8084) projected
  line L568 (-1.5661, 1.8084) -> (-1.5627, 1.7947) projected
  line L569 (-1.5627, 1.7947) -> (-1.5588, 1.7814) projected
  line L570 (-1.5588, 1.7814) -> (-1.5543, 1.7685) projected
  line L571 (-1.5543, 1.7685) -> (-1.5518, 1.7622) projected
  line L572 (-1.5518, 1.7622) -> (-1.5505, 1.7591) projected
  line L573 (-1.5505, 1.7591) -> (-1.5492, 1.7561) projected
  line L574 (-1.5492, 1.7561) -> (-1.5936, 1.7218) projected
  line L575 (-1.5936, 1.7218) -> (-1.5962, 1.7239) projected
  line L576 (-1.5962, 1.7239) -> (-1.5989, 1.7259) projected
  line L577 (-1.5989, 1.7259) -> (-1.6043, 1.7299) projected
  line L578 (-1.6043, 1.7299) -> (-1.6157, 1.7375) projected
  line L579 (-1.6157, 1.7375) -> (-1.6276, 1.7447) projected
  line L580 (-1.6276, 1.7447) -> (-1.6399, 1.7515) projected
  line L581 (-1.6399, 1.7515) -> (-1.6526, 1.7578) projected
  line L582 (-1.6526, 1.7578) -> (-1.6658, 1.7638) projected
  line L583 (-1.6658, 1.7638) -> (-1.7038, 1.7289) projected
  line L584 (-1.7038, 1.7289) -> (-1.699, 1.7153) projected
  line L585 (-1.699, 1.7153) -> (-1.6938, 1.7021) projected
  line L586 (-1.6938, 1.7021) -> (-1.6881, 1.6892) projected
  line L587 (-1.6881, 1.6892) -> (-1.682, 1.6768) projected
  line L588 (-1.682, 1.6768) -> (-1.6754, 1.6648) projected
  line L589 (-1.6754, 1.6648) -> (-1.6718, 1.659) projected
  line L590 (-1.6718, 1.659) -> (-1.67, 1.6562) projected
  line L591 (-1.67, 1.6562) -> (-1.6682, 1.6534) projected
  line L592 (-1.6682, 1.6534) -> (-1.7062, 1.6121) projected
  line L593 (-1.7062, 1.6121) -> (-1.7091, 1.6137) projected
  line L594 (-1.7091, 1.6137) -> (-1.7121, 1.6153) projected
  line L595 (-1.7121, 1.6153) -> (-1.7181, 1.6183) projected
  line L596 (-1.7181, 1.6183) -> (-1.7306, 1.6239) projected
  line L597 (-1.7306, 1.6239) -> (-1.7435, 1.629) projected
  line L598 (-1.7435, 1.629) -> (-1.7568, 1.6335) projected
  line L599 (-1.7568, 1.6335) -> (-1.7705, 1.6376) projected
  line L600 (-1.7705, 1.6376) -> (-1.7844, 1.6413) projected
  line L601 (-1.7844, 1.6413) -> (-1.816, 1.6005) projected
  line L602 (-1.816, 1.6005) -> (-1.809, 1.5879) projected
  line L603 (-1.809, 1.5879) -> (-1.8016, 1.5757) projected
  line L604 (-1.8016, 1.5757) -> (-1.7938, 1.564) projected
  line L605 (-1.7938, 1.564) -> (-1.7857, 1.5528) projected
  line L606 (-1.7857, 1.5528) -> (-1.7771, 1.5421) projected
  line L607 (-1.7771, 1.5421) -> (-1.7727, 1.537) projected
  line L608 (-1.7727, 1.537) -> (-1.7704, 1.5345) projected
  line L609 (-1.7704, 1.5345) -> (-1.7682, 1.5321) projected
  line L610 (-1.7682, 1.5321) -> (-1.7986, 1.485) projected
  line L611 (-1.7986, 1.485) -> (-1.8018, 1.486) projected
  line L612 (-1.8018, 1.486) -> (-1.805, 1.4871) projected
  line L613 (-1.805, 1.4871) -> (-1.8115, 1.489) projected
  line L614 (-1.8115, 1.489) -> (-1.8247, 1.4924) projected
  line L615 (-1.8247, 1.4924) -> (-1.8383, 1.4953) projected
  line L616 (-1.8383, 1.4953) -> (-1.8522, 1.4975) projected
  line L617 (-1.8522, 1.4975) -> (-1.8663, 1.4993) projected
  line L618 (-1.8663, 1.4993) -> (-1.8807, 1.5005) projected
  line L619 (-1.8807, 1.5005) -> (-1.9049, 1.455) projected
  line L620 (-1.9049, 1.455) -> (-1.8958, 1.4437) projected
  line L621 (-1.8958, 1.4437) -> (-1.8865, 1.433) projected
  line L622 (-1.8865, 1.433) -> (-1.8769, 1.4227) projected
  line L623 (-1.8769, 1.4227) -> (-1.867, 1.4131) projected
  line L624 (-1.867, 1.4131) -> (-1.8567, 1.404) projected
  line L625 (-1.8567, 1.404) -> (-1.8515, 1.3997) projected
  line L626 (-1.8515, 1.3997) -> (-1.8488, 1.3976) projected
  line L627 (-1.8488, 1.3976) -> (-1.8462, 1.3956) projected
  line L628 (-1.8462, 1.3956) -> (-1.8682, 1.344) projected
  line L629 (-1.8682, 1.344) -> (-1.8715, 1.3446) projected
  line L630 (-1.8715, 1.3446) -> (-1.8749, 1.345) projected
  line L631 (-1.8749, 1.345) -> (-1.8816, 1.3459) projected
  line L632 (-1.8816, 1.3459) -> (-1.8952, 1.347) projected
  line L633 (-1.8952, 1.347) -> (-1.9091, 1.3475) projected
  line L634 (-1.9091, 1.3475) -> (-1.9231, 1.3474) projected
  line L635 (-1.9231, 1.3474) -> (-1.9374, 1.3467) projected
  line L636 (-1.9374, 1.3467) -> (-1.9517, 1.3455) projected
  line L637 (-1.9517, 1.3455) -> (-1.9679, 1.2965) projected
  line L638 (-1.9679, 1.2965) -> (-1.9571, 1.287) projected
  line L639 (-1.9571, 1.287) -> (-1.9461, 1.278) projected
  line L640 (-1.9461, 1.278) -> (-1.9349, 1.2695) projected
  line L641 (-1.9349, 1.2695) -> (-1.9234, 1.2616) projected
  line L642 (-1.9234, 1.2616) -> (-1.9118, 1.2544) projected
  line L643 (-1.9118, 1.2544) -> (-1.9059, 1.251) projected
  line L644 (-1.9059, 1.251) -> (-1.903, 1.2495) projected
  line L645 (-1.903, 1.2495) -> (-1.9, 1.2479) projected
  line L646 (-1.9, 1.2479) -> (-1.913, 1.1933) projected
  line L647 (-1.913, 1.1933) -> (-1.9164, 1.1933) projected
  line L648 (-1.9164, 1.1933) -> (-1.9197, 1.1932) projected
  line L649 (-1.9197, 1.1932) -> (-1.9265, 1.1929) projected
  line L650 (-1.9265, 1.1929) -> (-1.9401, 1.1917) projected
  line L651 (-1.9401, 1.1917) -> (-1.9539, 1.1898) projected
  line L652 (-1.9539, 1.1898) -> (-1.9677, 1.1874) projected
  line L653 (-1.9677, 1.1874) -> (-1.9816, 1.1843) projected
  line L654 (-1.9816, 1.1843) -> (-1.9956, 1.1807) projected
  line L655 (-1.9956, 1.1807) -> (-2.0033, 1.1297) projected
  line L656 (-2.0033, 1.1297) -> (-1.991, 1.1221) projected
  line L657 (-1.991, 1.1221) -> (-1.9786, 1.1151) projected
  line L658 (-1.9786, 1.1151) -> (-1.9661, 1.1086) projected
  line L659 (-1.9661, 1.1086) -> (-1.9535, 1.1028) projected
  line L660 (-1.9535, 1.1028) -> (-1.9408, 1.0976) projected
  line L661 (-1.9408, 1.0976) -> (-1.9345, 1.0953) projected
  line L662 (-1.9345, 1.0953) -> (-1.9313, 1.0943) projected
  line L663 (-1.9313, 1.0943) -> (-1.9281, 1.0933) projected
  line L664 (-1.9281, 1.0933) -> (-1.9317, 1.0373) projected
  line L665 (-1.9317, 1.0373) -> (-1.935, 1.0367) projected
  circle A0 centre (-1.0054, 1.0054) radius 0.13 projected
  point P0 (0, 0)
body "Solid1"
